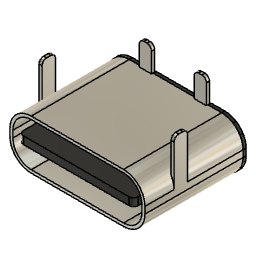
USB type C female 2P (Autodesk Fusion 360 design; units mm, degrees)
Autodesk Fusion 360 part; units mm, degrees
sketch "Sketch1" plane through (0, 0, 0) normal (0, 1, 0) x (1, 0, 0)
  line L0 (0.1, -0.1) -> (8.55, -0.1) construction
  line L1 (8.55, -0.1) -> (8.55, -2.94) construction
  line L2 (8.55, -2.94) -> (0.1, -2.94) construction
  line L3 (0.1, -2.94) -> (0.1, -0.1) construction
  line L4 (-0.1, 0.1) -> (8.75, 0.1)
  line L5 (8.75, 0.1) -> (8.75, -3.14)
  line L6 (8.75, -3.14) -> (-0.1, -3.14)
  line L7 (-0.1, -3.14) -> (-0.1, 0.1)
  line L8 (0, 0) -> (8.65, 0) construction
  line L9 (8.65, 0) -> (8.65, -3.04) construction
  line L10 (8.65, -3.04) -> (0, -3.04) construction
  line L11 (0, -3.04) -> (0, 0) construction
  dimension "d4" = -0.2
  dimension "d5" = -0.1
extrude "Extrude1" add sketch "Sketch1" along normal blind 6.43 makes body 1
fillet "Fillet1" radius 1.4 4 edges at (8.75, 3.215, 3.14) (8.75, 3.215, -0.1) (-0.1, 3.215, 3.14) (-0.1, 3.215, -0.1) on bodies 1
sketch "Sketch2" plane through (0, 0, 0) normal (0, -1, 0) x (1, 0, 0)
  arc A0 (-0.1, 1.3) -> (1.3, -0.1) centre (1.3, 1.3) ccw
  line L0 (1.3, -0.1) -> (7.35, -0.1)
  arc A1 (7.35, -0.1) -> (8.75, 1.3) centre (7.35, 1.3) ccw
  line L1 (8.75, 1.3) -> (8.75, 1.74)
  arc A2 (8.75, 1.74) -> (7.35, 3.14) centre (7.35, 1.74) ccw
  line L2 (7.35, 3.14) -> (1.3, 3.14)
  arc A3 (1.3, 3.14) -> (-0.1, 1.74) centre (1.3, 1.74) ccw
  line L3 (-0.1, 1.74) -> (-0.1, 1.3)
  line L4 (0.1, 1.74) -> (0.1, 1.3)
  arc A4 (0.1, 1.3) -> (1.3, 0.1) centre (1.3, 1.3) ccw
  line L5 (1.3, 0.1) -> (7.35, 0.1)
  arc A5 (7.35, 0.1) -> (8.55, 1.3) centre (7.35, 1.3) ccw
  line L6 (8.55, 1.3) -> (8.55, 1.74)
  arc A6 (8.55, 1.74) -> (7.35, 2.94) centre (7.35, 1.74) ccw
  line L7 (7.35, 2.94) -> (1.3, 2.94)
  arc A7 (1.3, 2.94) -> (0.1, 1.74) centre (1.3, 1.74) ccw
  dimension "d10" = -0.2
extrude "Extrude2" cut sketch "Sketch2" against normal blind 6.43 contours L4 A4 L5 A5 L6 A6 L7 A7 bodies 1
sketch "Sketch3" plane through (0, 6.43, 0) normal (0, 1, 0) x (-1, 0, 0)
  line L0 (-0.1, 1.74) -> (-0.1, 1.3)
  arc A0 (-1.3, 0.1) -> (-0.1, 1.3) centre (-1.3, 1.3) ccw
  line L1 (-1.3, 0.1) -> (-7.35, 0.1)
  arc A1 (-8.55, 1.3) -> (-7.35, 0.1) centre (-7.35, 1.3) ccw
  line L2 (-8.55, 1.3) -> (-8.55, 1.74)
  arc A2 (-7.35, 2.94) -> (-8.55, 1.74) centre (-7.35, 1.74) ccw
  line L3 (-7.35, 2.94) -> (-1.3, 2.94)
  arc A3 (-0.1, 1.74) -> (-1.3, 2.94) centre (-1.3, 1.74) ccw
  arc A4 (-1.3, -0.1) -> (0.1, 1.3) centre (-1.3, 1.3) ccw
  line L4 (0.1, 1.3) -> (0.1, 1.74)
  arc A5 (0.1, 1.74) -> (-1.3, 3.14) centre (-1.3, 1.74) ccw
  line L5 (-1.3, 3.14) -> (-7.35, 3.14)
  arc A6 (-7.35, 3.14) -> (-8.75, 1.74) centre (-7.35, 1.74) ccw
  line L6 (-8.75, 1.74) -> (-8.75, 1.3)
  arc A7 (-8.75, 1.3) -> (-7.35, -0.1) centre (-7.35, 1.3) ccw
  line L7 (-7.35, -0.1) -> (-1.3, -0.1)
  line L8 (-7.35, 3.14) -> (-1.3, 3.14)
  line L9 (0.1, 1.74) -> (0.1, 1.3)
  line L10 (-1.3, -0.1) -> (-7.35, -0.1)
  line L11 (-8.75, 1.3) -> (-8.75, 1.74)
  spline S0 degree 5 poles (-7.35, -0.1) (-7.4476, -0.1) (-7.6354, -0.0851) (-7.8944, -0.0183) (-8.1972, 0.1488) (-8.5012, 0.4528) (-8.6683, 0.7556) (-8.7351, 1.0146) (-8.75, 1.2024) (-8.75, 1.3) knots 0 0 0 0 0 0 0.2 0.4 0.6 0.8 1 1 1 1 1 1
  spline S1 degree 5 poles (-8.75, 1.74) (-8.75, 1.8376) (-8.7351, 2.0254) (-8.6683, 2.2844) (-8.5012, 2.5872) (-8.1972, 2.8912) (-7.8944, 3.0583) (-7.6354, 3.1251) (-7.4476, 3.14) (-7.35, 3.14) knots 0 0 0 0 0 0 0.2 0.4 0.6 0.8 1 1 1 1 1 1
  spline S2 degree 5 poles (-1.3, -0.1) (-1.2024, -0.1) (-1.0146, -0.0851) (-0.7556, -0.0183) (-0.4528, 0.1488) (-0.1488, 0.4528) (0.0183, 0.7556) (0.0851, 1.0146) (0.1, 1.2024) (0.1, 1.3) knots 0 0 0 0 0 0 0.2 0.4 0.6 0.8 1 1 1 1 1 1
  spline S3 degree 5 poles (0.1, 1.74) (0.1, 1.8376) (0.0851, 2.0254) (0.0183, 2.2844) (-0.1488, 2.5872) (-0.4528, 2.8912) (-0.7556, 3.0583) (-1.0146, 3.1251) (-1.2024, 3.14) (-1.3, 3.14) knots 0 0 0 0 0 0 0.2 0.4 0.6 0.8 1 1 1 1 1 1
  constraint horizontal L8
  constraint vertical L9
  constraint horizontal L10
  constraint vertical L11
  constraint coincident A7.end L7.start
  constraint coincident L6.end A7.start
  constraint coincident A6.end L6.start
  constraint coincident L5.end A6.start
  constraint coincident A4.start L7.end
  constraint coincident A4.end L4.start
  constraint coincident L4.end A5.start
  constraint coincident A5.end L5.start
extrude "Extrude3" add sketch "Sketch3" along normal blind 0.2 separate body contours L0 A0 L1 A1 L2 A2 L3 A3 | A4 L4 A5 L5 A6 L6 A7 L7 L8 L9 L10 L11 S0 S1 S2 S3 makes body 2
sketch "Sketch4" plane through (0, 0, 0) normal (0, 1, 0) x (1, 0, 0)
  line L0 (8.6991, -3.1025) -> (0, 0) construction
  line L1 (-0.1103, -3.1118) -> (8.7397, 0.1282) construction
  line L2 (4.2496, -1.5156) -> (4.3035, 0.7511) construction
  line L3 (8.0099, -1.2656) -> (0.4893, -1.2656)
  line L4 (0.4893, -1.2656) -> (0.4893, -1.7656)
  line L5 (0.4893, -1.7656) -> (8.0099, -1.7656)
  line L6 (8.0099, -1.7656) -> (8.0099, -1.2656)
  line L7 (8.0099, -1.2656) -> (0.4893, -1.7656) construction
  line L8 (0.4893, -1.2656) -> (8.0099, -1.7656) construction
  point P0 (4.2496, -1.5156)
  dimension "d15" = 0.5
  constraint coincident L0.end origin
  constraint coincident L0 P0
  constraint coincident L1 P0
  constraint horizontal L3
  constraint perpendicular L3 L4
  constraint parallel L3 L5
  constraint parallel L4 L6
  constraint coincident L7 P0
  constraint coincident L8 P0
  constraint coincident P0 L2.start
  measures "d15" distance of L3.end L4.end
extrude "Extrude4" add sketch "Sketch4" along normal blind 6.43 separate body makes body 3
fillet "Fillet2" radius 0.3 2 edges at (8.0099, 0, 1.5156) (0.4893, 0, 1.5156) on bodies 3
sketch "Sketch5" plane through (0, 0, 3.14) normal (0, 0, 1) x (-1, 0, 0)
  line L0 (-1.3, -6.43) -> (-1.3, 0)
  line L1 (-1.3, 0) -> (-7.35, 0)
  line L2 (-7.35, 0) -> (-7.35, -6.43)
  line L3 (-7.35, -6.43) -> (-1.3, -6.43)
  line L4 (-4.25, 0.05) -> (-4.25, -8) construction
  line L5 (0, 0) -> (-8.7598, -6.43) construction
  line L6 (-4.25, -6.43) -> (-2.45, -6.43) construction
  line L7 (-4.25, -6.43) -> (-6.05, -6.43) construction
  line L8 (-5.65, -6.53) -> (-6.45, -6.53)
  line L9 (-6.45, -6.53) -> (-6.45, -6.33)
  line L10 (-6.45, -6.33) -> (-5.65, -6.33)
  line L11 (-5.65, -6.33) -> (-5.65, -6.53)
  line L12 (-5.65, -6.53) -> (-6.45, -6.33) construction
  line L13 (-6.45, -6.53) -> (-5.65, -6.33) construction
  line L14 (-2.05, -6.53) -> (-2.85, -6.53)
  line L15 (-2.85, -6.53) -> (-2.85, -6.33)
  line L16 (-2.85, -6.33) -> (-2.05, -6.33)
  line L17 (-2.05, -6.33) -> (-2.05, -6.53)
  line L18 (-2.05, -6.53) -> (-2.85, -6.33) construction
  line L19 (-2.85, -6.53) -> (-2.05, -6.33) construction
  line L20 (-6.45, -6.53) -> (-6.45, -6.63)
  line L21 (-6.45, -6.63) -> (-5.65, -6.63)
  line L22 (-5.65, -6.63) -> (-5.65, -6.53)
  line L23 (-2.85, -6.53) -> (-2.85, -6.63)
  line L24 (-2.85, -6.63) -> (-2.05, -6.63)
  line L25 (-2.05, -6.63) -> (-2.05, -6.53)
  point P0 (-6.05, -6.43)
  point P1 (-2.45, -6.43)
  dimension "d20" = 1.8
  dimension "d21" = 1.8
  dimension "d22" = 0.8
  dimension "d23" = 0.2
  dimension "d24" = 0.8
  dimension "d25" = 0.2
  constraint perpendicular L3 L4
  constraint coincident L5.start origin
  constraint coincident L4 L6.start
  constraint coincident L3 L6.start
  constraint perpendicular L4 L6
  constraint perpendicular L4 L7
  constraint horizontal L8
  constraint perpendicular L8 L9
  constraint parallel L8 L10
  constraint parallel L9 L11
  constraint coincident L12 P0
  constraint coincident L13 P0
  constraint coincident P0 L7.end
  constraint horizontal L14
  constraint perpendicular L14 L15
  constraint parallel L14 L16
  constraint parallel L15 L17
  constraint coincident L18 P1
  constraint coincident L19 P1
  constraint coincident P1 L6.end
  constraint perpendicular L8 L20
  constraint perpendicular L11 L21
  constraint perpendicular L8 L22
  constraint perpendicular L14 L23
  constraint perpendicular L17 L24
  constraint perpendicular L14 L25
  measures "d20" distance of L6.start P1
  measures "d21" distance of L6.start P0
  measures "d22" distance of L9.end L10.end
  measures "d23" distance of L8.end L9.end
  measures "d24" distance of L15.end L16.end
  measures "d25" distance of L14.end L15.end
extrude "Extrude5" add sketch "Sketch5" along normal blind 1.6 separate body contours L3 L14 L15 L17 | L3 L15 L16 L17 | L3 L8 L9 L11 | L3 L9 L10 L11 makes body 4 at (6.1833, 6.33, 3.6733) makes body 5 at (2.3167, 6.53, 3.6733)
fillet "Fillet3" radius 0.3 4 edges at (5.65, 6.43, 4.74) (6.45, 6.43, 4.74) (2.85, 6.43, 4.74) (2.05, 6.43, 4.74) on bodies 4 5
extrude "Extrude6" cut sketch "Sketch5" against normal blind 3.3 contours L14 L23 L24 L25 | L8 L20 L21 L22 bodies 2
sketch "Sketch6" plane through (0, 0, 3.14) normal (0, 0, 1) x (-1, 0, 0)
  line L0 (-1.3, -6.43) -> (-1.3, 0)
  line L1 (-1.3, 0) -> (-7.35, 0)
  line L2 (-7.35, 0) -> (-7.35, -6.43)
  line L3 (-7.35, -6.43) -> (-1.3, -6.43)
  line L4 (1.0089, -6.43) -> (-10, -6.43) construction
  line L5 (0.1, -6.7) -> (0.1, 0.5) construction
  line L6 (-8.75, -6.7) -> (-8.75, 0.5) construction
  line L7 (0.1, -6.43) -> (0.1, -2.35) construction
  line L8 (0.1, -2.35) -> (-8.75, -2.35) construction
  line L9 (-8.55, -2.79) -> (-8.75, -2.79)
  line L10 (-8.75, -2.79) -> (-8.75, -1.91)
  line L11 (-8.75, -1.91) -> (-8.55, -1.91)
  line L12 (-8.55, -1.91) -> (-8.55, -2.79)
  line L13 (-8.75, -2.79) -> (-8.55, -1.91) construction
  line L14 (-8.55, -2.79) -> (-8.75, -1.91) construction
  line L15 (-0.1, -2.79) -> (0.1, -1.91) construction
  line L16 (0, -2.35) -> (0.1, -2.35) construction
  line L17 (-0.1, -2.79) -> (-0.1, -1.91)
  line L18 (-0.1, -1.91) -> (0.1, -1.91)
  line L19 (0.1, -1.91) -> (0.1, -2.79)
  line L20 (0.1, -2.79) -> (-0.1, -2.79)
  line L21 (0.1, -2.79) -> (-0.1, -1.91) construction
  line L22 (-8.65, -2.35) -> (-8.75, -2.35) construction
  dimension "d32" = 4.08
  dimension "d33" = 0.2
  dimension "d34" = 0.88
  dimension "d35" = 0.2
  dimension "d36" = 0.88
  constraint parallel L3 L4
  constraint perpendicular L4 L5
  constraint perpendicular L4 L6
  constraint coincident L4 L7.start
  constraint coincident L5 L7.start
  constraint perpendicular L4 L7
  constraint coincident L6 L8.end
  constraint perpendicular L6 L8
  constraint horizontal L9
  constraint vertical L10
  constraint horizontal L11
  constraint vertical L12
  constraint horizontal L20
  constraint vertical L17
  constraint horizontal L18
  constraint vertical L19
  constraint midpoint L16.start L15
  constraint midpoint L7.end L19
  constraint midpoint L14 L22.start
  constraint midpoint L10 L8.end
  measures "d32" distance of L7.start L7.end
  measures "d33" distance of L9.start L9.end
  measures "d34" distance of L9.start L11.end
  measures "d35" distance of L19.end L15.start
  measures "d36" distance of L15.end L19.end
extrude "Extrude7" add sketch "Sketch6" along normal blind 1.6 separate body contours L9 L10 L11 L12 | L17 L18 L19 L20 makes body 6 at (8.75, 2.4967, 3.6733) makes body 7 at (0.1, 2.4967, 3.6733)
fillet "Fillet4" radius 0.3 4 edges at (8.65, 2.79, 4.74) (8.65, 1.91, 4.74) (0, 1.91, 4.74) (0, 2.79, 4.74) on bodies 6 7
extrude "Extrude8" add 2 faces at (0.0333, 2.2033, 3.14) (8.6833, 2.2033, 3.14) along direction (0, 0, -1) blind 1.4 on bodies 6 7 bodies 1 2 3 4 5 7 6
